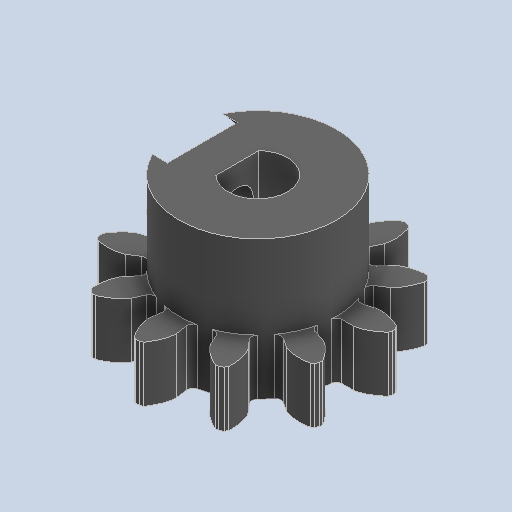
# Autodesk Inventor part: screw_gear_under_12
Saved by Autodesk Inventor 2024.1 (Build 281209000, 209)
## iProperties
Created: 2025-01-10
Part Number: screw_gear_under_12
Material: 一般
Document SubType Name: Modeling
Designer: hibik
Density: 1 g/cm^3
Appearance: 既定
Author: hibik
Autodesk Inventor part; units mm, degrees
ref_plane "XZ Plane" through (0, 0, 0) normal (0, 1, 0) x (-1, 0, 0)
sketch "スケッチ1" plane through (0, 0, 0) normal (0, 1, 0) x (-1, 0, 0)
  circle A0 centre (0, 0) radius 5.5 construction
  circle A1 centre (0, 0) radius 5.1683 construction
  line L0 (0, 0) -> (0.7355, -5.1157)
  line L1 (0, -10.5007) -> (0, 8.7501) projected
  dimension "d1" = 10.3366
  dimension "d0" = 11
  dimension "d4" = 8.182
  constraints: 3 coincident, 2 end point, 1 centre point, 7 other
  measures "d0" diameter of A0
  measures "d4" angle of L1 L0
sketch "スケッチ2" plane through (0, 0, 0) normal (0, 1, 0) x (-1, 0, 0)
  circle A0 centre (0, 0) radius 6.5
  dimension "d5" = 13
  constraints: 1 centre point, 1 coincident
  measures "d5" diameter of A0
extrude "押し出し1" add sketch "スケッチ2" along normal blind 3
sketch "スケッチ3" plane through (0, 3, 0) normal (0, 1, 0) x (1, 0, 0)
  line L0 (0, 0) -> (-0.7355, 5.1157) projected
  spline S0 degree 3 poles (-0.7355, 5.1157) (-0.7355, 5.1158) (-0.8126, 5.5427) (-1.3851, 6.0793) (-1.6608, 6.3379) (-2.0474, 6.6147) (-2.557, 6.8472) knots 0 0 0 0 0.674859 0.674859 0.674859 1 1 1 1 projected
  circle A0 centre (0, 0) radius 6.5 projected
  circle A1 centre (0, 0) radius 4.25
  line L1 (0, 10.7) -> (0, -9.95) projected
  point P0 (0, 4.25)
  point P1 (0, 6.5)
  point P2 (-1.6329, 6.2915)
  point P3 (-0.6048, 4.2067)
  dimension "d10" = 8.5
  constraints: 3 coincident, 1 centre point
  measures "d10" diameter of A1
extrude "押し出し2" cut sketch "スケッチ3" against normal through all contours L0 S0 A0 L1 A1 picked at (-0.2452, 5.2886)
fillet "フィレット1" radius 0.3 1 edges at (-0.6048, 1.5, -4.2067)
chamfer "面取り1" distance 0.1 angle 45 1 edges at (-1.6329, 1.5, -6.2915)
mirror "ミラー1" about plane through (0, 3, -6.5) normal (-1, 0, 0) of "押し出し2", "フィレット1", "面取り1"
pattern_circular "円形状パターン1" count 11 over 360 about axis through (0, -10, 0) along (0, 1, 0) of "押し出し2", "フィレット1", "面取り1", "ミラー1"
sketch "スケッチ4" plane through (0, 3, 0) normal (0, 1, 0) x (1, 0, 0)
  circle A0 centre (0, 0) radius 4.25
  dimension "d20" = 8.5
  constraints: 1 centre point, 1 coincident
  measures "d20" diameter of A0
extrude "押し出し3" add sketch "スケッチ4" along normal blind 4.5
sketch "スケッチ5" plane through (0, 7.5, 0) normal (0, 1, 0) x (1, 0, 0)
  circle A0 centre (0, 0) radius 1.6
  dimension "d23" = 3.2
  constraints: 1 centre point, 1 coincident
  measures "d23" diameter of A0
extrude "押し出し4" cut sketch "スケッチ5" against normal through all
sketch "スケッチ6" plane through (0, 0, 0) normal (0, -1, 0) x (1, 0, 0)
  circle A0 centre (0, 0) radius 3.05
  dimension "d26" = 6.1
  constraints: 1 centre point, 1 coincident
  measures "d26" diameter of A0
extrude "押し出し5" cut sketch "スケッチ6" against normal blind 2.5
sketch "スケッチ7" plane through (0, 0, 0) normal (1, 0, 0) x (0, 1, 0)
  line L0 (7.5, -4.25) -> (7.5, 4.25) projected
  line L1 (2.5, -3.05) -> (2.5, 3.05) projected
  circle A0 centre (5.5, 0) radius 0.85
  point P0 (0, 0)
  point P1 (7.5, 0)
  dimension "d29" = 1.7
  dimension "d40" = 2
  constraints: 1 centre point, 1 coincident, 1 horizontal alignment, 1 midpoint
  measures "d29" diameter of A0
  measures "d40" distance from line of L0 A0.centre
extrude "押し出し6" cut sketch "スケッチ7" against normal through all
ref_plane "作業平面1" through (-3, 0, 0) normal (1, 0, 0) x (0, 1, 0)
sketch "スケッチ8" plane through (-3, 0, 0) normal (1, 0, 0) x (0, 1, 0)
  circle A0 centre (5.5, 0) radius 2.75
  line L0 (7.5, 1.6) -> (7.5, -1.6) projected
  line L1 (2.5, 1.6) -> (2.5, -1.6) projected
  line L2 (2.5, -3.05) -> (2.5, 3.05) projected
  line L3 (2.5, 1.6) -> (2.5, -1.6) projected
  point P0 (0, 0)
  point P1 (2.5, 1.1456)
  point P2 (2.5, -1.1456)
  point P3 (7.5, 0)
  dimension "d33" = 5.5
  dimension "d41" = 2
  constraints: 1 centre point, 1 coincident, 1 horizontal alignment, 1 midpoint, 3 other
  measures "d33" diameter of A0
  measures "d41" distance from line of L0 A0.centre
extrude "押し出し7" cut sketch "スケッチ8" against normal through all
ref_plane "作業平面2" through (-1.1, 0, 0) normal (1, 0, 0) x (0, 1, 0)
sketch "スケッチ9" plane through (-1.1, 0, 0) normal (1, 0, 0) x (0, 1, 0)
  line L0 (7.5, -4.25) -> (7.5, 4.25) projected
  line L1 (2.5, -3.05) -> (2.5, 3.05) projected
  line L2 (2.5, -1.5) -> (7.5, -1.5)
  line L3 (7.5, -1.5) -> (7.5, 1.5)
  line L4 (7.5, 1.5) -> (2.5, 1.5)
  line L5 (2.5, 1.5) -> (2.5, -1.5)
  line L6 (2.5, 0) -> (7.5, 0)
  spline S0 degree 5 poles (6.35, 0) (6.35, 0.1675) (6.3085, 0.3349) (6.2273, 0.4797) (6.1235, 0.5973) (5.914, 0.7501) (5.8179, 0.7993) (5.7147, 0.8329) (5.6074, 0.85) (5.3927, 0.85) (5.2855, 0.8329) (5.1823, 0.7994) (5.0863, 0.7503) (4.9338, 0.6392) (4.8733, 0.5831) (4.8192, 0.5193) (4.7728, 0.4484) (4.7026, 0.3037) (4.6767, 0.2315) (4.6589, 0.1557) (4.65, 0.078) (4.65, -0.1675) (4.6915, -0.3349) (4.7727, -0.4797) (4.8765, -0.5973) (5.086, -0.7501) (5.1821, -0.7993) (5.2853, -0.8329) (5.3926, -0.85) (5.6073, -0.85) (5.7145, -0.8329) (5.8177, -0.7994) (5.9137, -0.7503) (6.0662, -0.6392) (6.1267, -0.5831) (6.1808, -0.5193) (6.2272, -0.4484) (6.2974, -0.3037) (6.3233, -0.2315) (6.3411, -0.1557) (6.35, -0.078) (6.35, 0) knots 0 0 0 0 0 0 0.146408 0.146408 0.146408 0.146408 0.250229 0.250229 0.250229 0.250229 0.353974 0.353974 0.353974 0.353974 0.432259 0.432259 0.432259 0.432259 0.500333 0.500333 0.500333 0.500333 0.646546 0.646546 0.646546 0.646546 0.750229 0.750229 0.750229 0.750229 0.853836 0.853836 0.853836 0.853836 0.932017 0.932017 0.932017 0.932017 1 1 1 1 1 1 projected
  line L7 (2.5, 1.6) -> (2.5, -1.6) projected
  line L8 (7.5, 1.6) -> (7.5, -1.6) projected
  point P0 (0, 0)
  point P1 (7.5, 1.8875)
  point P2 (7.5, -1.8875)
  point P3 (2.5, 1.5)
  dimension "d37" = 3
  constraints: 10 end point, 4 midpoint, 2 parallel, 2 perpendicular, 2 point on line, 1 horizontal, 2 other
  measures "d37" distance between parallel lines of L4 L2
extrude "押し出し8" add sketch "スケッチ9" against normal up to surface (1.9 mm away) contours L2 L1 L6 S0 L0 | L6 S0 L1 L4 L0
equation "\"module\" = 1"
